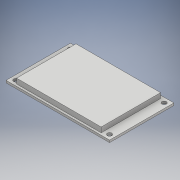
# Autodesk Inventor part: M024-ILI9328 data
Saved by Autodesk Inventor 2018 (Build 220112000, 112)
## iProperties
Created: 2019-04-02
Part Number: M024-ILI9328 data
Material: 一般
Document SubType Name: Modeling
Designer: rakur
Density: 1 g/cm^3
Appearance: 既定
Author: rakur
Autodesk Inventor part; units mm, degrees
ref_plane "YZ Plane" through (0, 0, 0) normal (1, 0, 0) x (0, 1, 0)
ref_plane "XZ Plane" through (0, 0, 0) normal (0, 1, 0) x (-1, 0, 0)
ref_plane "XY Plane" through (0, 0, 0) normal (0, 0, 1) x (1, 0, 0)
sketch "スケッチ1" plane through (0, 0, 0) normal (0, 0, 1) x (1, 0, 0)
  line L0 (0, 0) -> (74, 0)
  line L1 (74, 0) -> (74, 46)
  line L2 (74, 46) -> (0, 46)
  line L3 (0, 46) -> (0, 0)
  circle A0 centre (3.5, 42.5) radius 1.6
  circle A1 centre (3.5, 3.5) radius 1.6
  circle A2 centre (70.5, 3.5) radius 1.6
  circle A3 centre (70.5, 42.5) radius 1.6
  line L4 (5, 33) -> (2, 33)
  line L5 (2, 33) -> (2, 13)
  line L6 (2, 13) -> (5, 13)
  line L7 (5, 13) -> (5, 33)
  line L8 (6, 1.5) -> (66.5, 1.5)
  line L9 (66.5, 1.5) -> (66.5, 44)
  line L10 (66.5, 44) -> (6, 44)
  line L11 (6, 44) -> (6, 1.5)
  constraints: 24 end point, 6 parallel, 4 centre point, 3 horizontal, 3 perpendicular
extrude "押し出し1" add sketch "スケッチ1" along normal blind 1.6 contours L3 L2 L1 L0 | L7 L6 L5 L4 | L11 L10 L9 L8
sketch "スケッチ3" plane through (0, 0, 1.6) normal (0, 0, 1) x (1, 0, 0)
  line L0 (0, 0) -> (74, 0)
  line L1 (74, 0) -> (74, 46)
  line L2 (74, 46) -> (0, 46)
  line L3 (0, 46) -> (0, 0)
  circle A0 centre (3.5, 42.5) radius 1.6
  circle A1 centre (3.5, 3.5) radius 1.6
  circle A2 centre (70.5, 3.5) radius 1.6
  circle A3 centre (70.5, 42.5) radius 1.6
  line L4 (5, 33) -> (2, 33)
  line L5 (2, 33) -> (2, 13)
  line L6 (2, 13) -> (5, 13)
  line L7 (5, 13) -> (5, 33)
  line L8 (6, 1.5) -> (66.5, 1.5)
  line L9 (66.5, 1.5) -> (66.5, 44)
  line L10 (66.5, 44) -> (6, 44)
  line L11 (6, 44) -> (6, 1.5)
  constraints: 24 end point, 6 parallel, 4 centre point, 3 horizontal, 3 perpendicular
extrude "押し出し2" add sketch "スケッチ3" along normal blind 3.6 contours L11 L10 L9 L8
